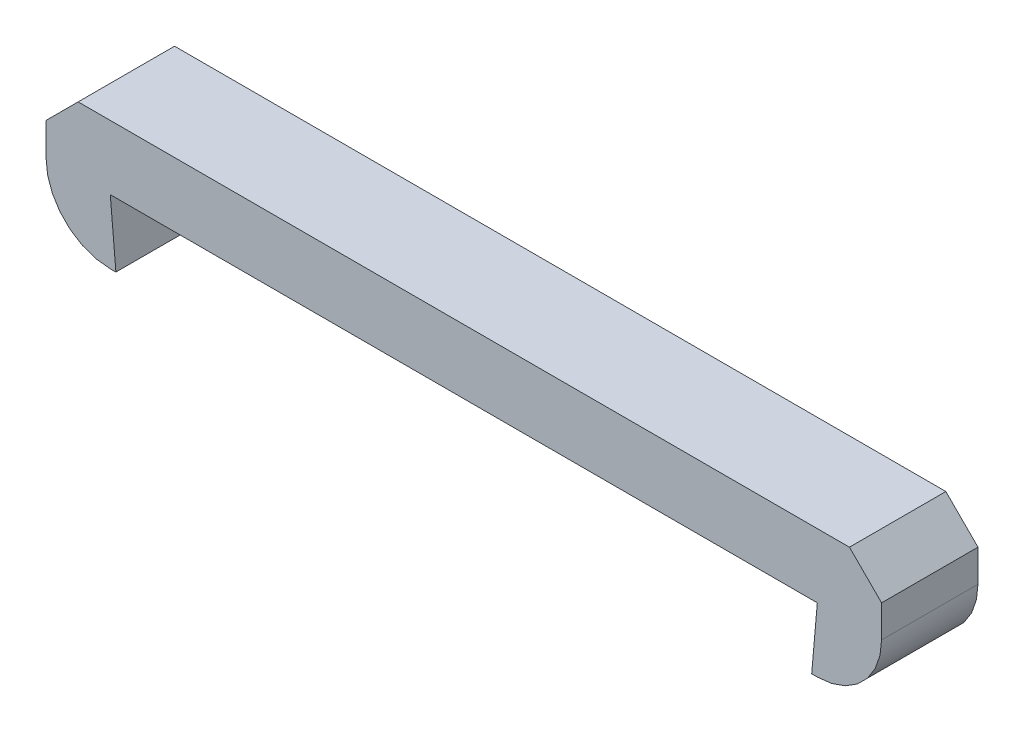
# Autodesk Inventor part: Clip
Saved by Autodesk Inventor 2024 (Build 280153000, 153)
## iProperties
Created: 2023-10-18
Part Number: Clip
Material: Generic
Document SubType Name: Modeling
Designer: Gurra
Density: 1 g/cm^3
Appearance: Default
Author: Gurra
Autodesk Inventor part; units mm, degrees
ref_plane "YZ Plane" through (0, 0, 0) normal (1, 0, 0) x (0, 1, 0)
ref_plane "XZ Plane" through (0, 0, 0) normal (0, 1, 0) x (-1, 0, 0)
ref_plane "XY Plane" through (0, 0, 0) normal (0, 0, 1) x (1, 0, 0)
sketch "Sketch2" plane through (0, 0, 0) normal (0, 0, 1) x (1, 0, 0)
  line L0 (0, 0) -> (-25, 0)
  line L1 (-25, 0) -> (-25, -2)
  line L2 (-25, -2) -> (0, -2)
  line L3 (0, -2) -> (0, 0)
  line L4 (-25.5, 0) -> (-23.5, 0)
  line L5 (-23.5, 0) -> (-23.5, -4)
  line L6 (-23.5, -4) -> (-25.5, -4)
  line L7 (-25.5, -4) -> (-25.5, 0)
  line L8 (0.5, 0) -> (-1.5, 0)
  line L9 (-1.5, 0) -> (-1.5, -4)
  line L10 (-1.5, -4) -> (0.5, -4)
  line L11 (0.5, -4) -> (0.5, 0)
  point P0 (-23.5, -2)
  point P1 (-1.5, -2)
  dimension "d0" = 25
  dimension "d1" = 2
  dimension "d2" = 2
  dimension "d3" = 4
  dimension "d4" = 2
  dimension "d5" = 4
  constraints: 24 end point, 6 parallel, 3 horizontal, 3 perpendicular
  measures "d0" distance of L2.end L1.end
  measures "d1" distance of L1.end L0.end
  measures "d2" distance of L5.end L6.end
  measures "d3" distance of L4.end L5.end
  measures "d4" distance of L10.end L9.end
  measures "d5" distance of L9.end L8.end
extrude "Extrusion1" add sketch "Sketch2" along normal blind 3
chamfer "Chamfer1" distance 1 angle 45 2 edges at (-25.5, 0, 1.5) (0.5, 0, 1.5)
draft "FaceDraft1" angle -5 pull direction (0, -1, 0) faces at (-23.5, -3.3333, 1) fixed edges at (-23.5, -2, 1.5)
draft "FaceDraft2" angle -5 pull direction (0, -1, 0) faces at (-1.5, -2.6667, 1) fixed edges at (-1.5, -2, 1.5)
fillet "Fillet1" radius 2 2 edges at (-25.5, -4, 1.5) (0.5, -4, 1.5)
body "Solid1"
